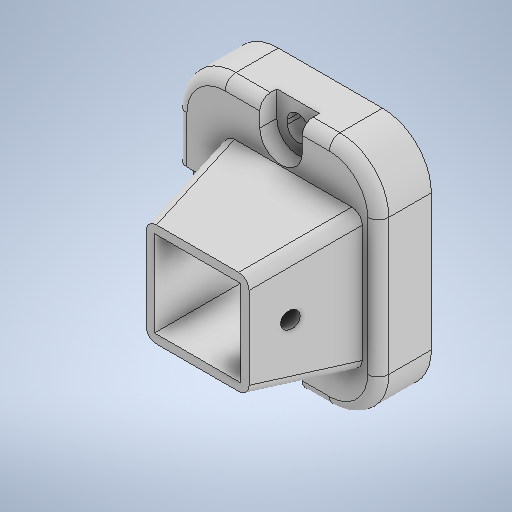
# Autodesk Inventor part: HD - 408 PERFIL ALUMINIO - ANCLAJE BASE DE COLUMNA 40X40
Saved by Autodesk Inventor 2025 (Build 290162000, 162)
## iProperties
Created: 2026-01-26
Part Number: HD - 408 PERFIL ALUMINIO - ANCLAJE BASE DE COLUMNA 40X40
Material: Generic
Document SubType Name: Modeling
Designer: Frank
Density: 1 g/cm^3
Appearance: Default
Author: Frank
Autodesk Inventor part; units mm, degrees
sketch "Sketch1" plane through (0, 0, 0) normal (0, 0, 1) x (1, 0, 0)
  line L0 (-72, 110) -> (-23, 110)
  line L1 (0, 87) -> (0, 23)
  line L2 (-23, 0) -> (-72, 0)
  line L3 (-95, 23) -> (-95, 87)
  arc A0 (-72, 110) -> (-95, 87) centre (-72, 87) ccw
  arc A1 (-95, 23) -> (-72, 0) centre (-72, 23) ccw
  arc A2 (-23, 0) -> (0, 23) centre (-23, 23) ccw
  arc A3 (0, 87) -> (-23, 110) centre (-23, 87) ccw
  point P0 (0, 0)
  point P1 (-95, 110)
  point P2 (0, 0)
  point P3 (0, 110)
  point P4 (-95, 0)
  dimension "d0" = 95
  dimension "d1" = 110
  dimension "d2" = 23
  constraints: 8 end point, 8 point on circle, 8 point on line, 8 tangent, 4 centre point, 3 equal radius, 2 parallel, 1 coincident, 1 horizontal, 1 perpendicular
  measures "d0" distance of point (-95, 110) point (0, 110)
  measures "d1" distance of point (-95, 0) point (-95, 110)
  measures "d2" radius of A0
extrude "Extrusion1" add sketch "Sketch1" against normal blind 25
fillet "Fillet1" radius 5 8 edges at (-47.5, 0, 0) (-6.7365, 6.7365, 0) (0, 55, 0) (-6.7365, 103.2635, 0) (-47.5, 110, 0) (-88.2635, 103.2635, 0) (-95, 55, 0) (-88.2635, 6.7365, 0)
sketch "Sketch2" plane through (0, 0, 0) normal (0, 0, 1) x (1, 0, 0)
  line L0 (-35.7103, 0) -> (-35.7103, 12)
  line L1 (-55.7103, 0) -> (-55.7103, 12)
  arc A0 (-35.7103, 12) -> (-55.7103, 12) centre (-45.7103, 12) ccw
  line L2 (-40.7103, 10) -> (-40.7103, 12)
  line L3 (-50.7103, 10) -> (-50.7103, 12)
  arc A1 (-40.7103, 12) -> (-50.7103, 12) centre (-45.7103, 12) ccw
  arc A2 (-50.7103, 10) -> (-40.7103, 10) centre (-45.7103, 10) ccw
  line L4 (-55.7103, 0) -> (-35.7103, 0)
  line L5 (-23, 0) -> (-72, 0) projected
  point P0 (0, 0)
  point P1 (-45.7103, 22)
  point P2 (-45.7103, 17)
  point P3 (-45.7103, 5)
  dimension "d5" = 20
  dimension "d9" = 5
  dimension "d11" = 10
  constraints: 10 end point, 9 point on circle, 6 tangent, 3 centre point, 2 vertical, 1 collinear
  measures "d5" distance between parallel lines of L1 L0
  measures "d9" distance of point (-45.71, 22) point (-45.71, 17)
  measures "d11" distance between parallel lines of L2 L3
extrude "Extrusion2" cut sketch "Sketch2" against normal blind 8
sketch "Sketch3" plane through (0, 0, 0) normal (0, 0, 1) x (1, 0, 0)
  line L0 (-40.7103, 10) -> (-40.7103, 12) projected
  line L1 (-40.7103, 12) -> (-40.7103, 10)
  arc A0 (-40.7103, 12) -> (-50.7103, 12) centre (-45.7103, 12) ccw projected
  line L2 (-50.7103, 12) -> (-50.7103, 10) projected
  line L3 (-50.7103, 12) -> (-50.7103, 10)
  arc A1 (-50.7103, 10) -> (-40.7103, 10) centre (-45.7103, 10) ccw projected
  point P0 (0, 0)
  constraints: 4 end point, 1 collinear, 1 vertical
extrude "Extrusion3" cut sketch "Sketch3" against normal through all
ref_plane "Work Plane1" through (-72, 55, -25) normal (0, -1, 0) x (1, 0, 0)
mirror "Mirror1" about plane through (-72, 55, -25) normal (0, -1, 0) of "Extrusion2"
mirror "Mirror2" about plane through (-72, 55, -25) normal (0, -1, 0) of "Extrusion3"
sketch "Sketch5" plane through (0, 0, 0) normal (0, 0, 1) x (1, 0, 0)
  line L0 (-95, 23) -> (-95, 87) projected
  line L1 (-95, 45) -> (-83, 45)
  line L2 (-83, 65) -> (-95, 65)
  line L3 (-95, 65) -> (-95, 45)
  line L4 (19, 55) -> (-114, 55) projected
  arc A0 (-83, 45) -> (-83, 65) centre (-83, 55) ccw
  line L5 (-83, 60) -> (-85, 60)
  line L6 (-85, 50) -> (-83, 50)
  arc A1 (-83, 50) -> (-83, 60) centre (-83, 55) ccw
  arc A2 (-85, 60) -> (-85, 50) centre (-85, 55) ccw
  line L7 (-90, 23) -> (-90, 87) projected
  point P0 (0, 0)
  point P1 (-73, 55)
  point P2 (-78, 55)
  point P3 (-90, 55)
  dimension "d21" = 20
  dimension "d22" = 10
  dimension "d23" = 10
  dimension "d24" = 5
  dimension "d25" = 5
  dimension "d26" = 5
  dimension "d27" = 12
  constraints: 10 end point, 9 point on circle, 6 tangent, 3 centre point, 2 horizontal, 2 parallel, 1 point on line
  measures "d21" distance between parallel lines of L2 L1
  measures "d22" distance between parallel lines of L1 L4
  measures "d23" distance between parallel lines of L6 L5
  measures "d24" distance between parallel lines of L1 L6
  measures "d25" distance of point (-73, 55) point (-78, 55)
  measures "d26" distance from line of L0 point (-90, 55)
  measures "d27" distance from line of L7 point (-78, 55)
extrude "Extrusion4" cut sketch "Sketch5" against normal blind 8 contours L0 L4 L7 L1 | L0 L2 L7 L4 | L7 A2 L6 A1 L4 A0 L1 | L7 L2 A0 L4 A1 L5 A2
sketch "Sketch6" plane through (0, 0, 0) normal (0, 0, 1) x (1, 0, 0)
  arc A0 (-83, 50) -> (-83, 60) centre (-83, 55) ccw projected
  line L0 (-83, 60) -> (-85, 60) projected
  line L1 (-83, 60) -> (-85, 60)
  line L2 (-85, 50) -> (-83, 50) projected
  line L3 (-83, 50) -> (-85, 50)
  arc A1 (-85, 60) -> (-85, 50) centre (-85, 55) ccw projected
  point P0 (0, 0)
  constraints: 4 end point, 1 collinear, 1 horizontal
extrude "Extrusion5" cut sketch "Sketch6" against normal through all
sketch "Sketch9" plane through (0, 0, 0) normal (0, 0, 1) x (1, 0, 0)
  line L0 (-72.5, 22.5) -> (-7.5, 22.5)
  line L1 (-7.5, 22.5) -> (-7.5, 87.5)
  line L2 (-7.5, 87.5) -> (-72.5, 87.5)
  line L3 (-72.5, 87.5) -> (-72.5, 22.5)
  line L4 (-5, 87) -> (-5, 23) projected
  line L5 (-72, 0) -> (-55.7103, 0) projected
  point P0 (0, 0)
  point P1 (-40, 22.5)
  dimension "d42" = 65
  dimension "d43" = 65
  dimension "d44" = 2.5
  dimension "d45" = 22.5
  constraints: 8 end point, 2 parallel, 1 horizontal, 1 midpoint, 1 perpendicular
  measures "d42" distance of L2.end L0.start
  measures "d43" distance of L0.start L0.end
  measures "d44" distance between parallel lines of L4 L1
  measures "d45" distance from line of L5 point (-40, 22.5)
ref_plane "Work Plane3" through (0, 0, 45) normal (0, 0, 1) x (1, 0, 0)
sketch "Sketch10" plane through (0, 0, 45) normal (0, 0, 1) x (1, 0, 0)
  line L0 (-64.25, 30.75) -> (-15.75, 30.75)
  line L1 (-15.75, 30.75) -> (-15.75, 79.25)
  line L2 (-15.75, 79.25) -> (-64.25, 79.25)
  line L3 (-64.25, 79.25) -> (-64.25, 30.75)
  line L4 (0, 23) -> (0, 87) projected
  line L5 (-35.7103, 0) -> (-55.7103, 0) projected
  line L6 (-55.7103, 110) -> (-35.7103, 110) projected
  line L7 (-95, 45) -> (-95, 65) projected
  point P0 (0, 0)
  dimension "d47" = 48.5
  dimension "d48" = 48.5
  dimension "d51" = 30.75
  dimension "d52" = 30.75
  dimension "d53" = 30.75
  constraints: 8 end point, 2 parallel, 1 horizontal, 1 perpendicular
  measures "d47" distance of L2.end L0.start
  measures "d48" distance of L0.start L0.end
  measures "d51" distance between parallel lines of L5 L0
  measures "d52" distance between parallel lines of L6 L2
  measures "d53" distance between parallel lines of L7 L3
loft "Loft1" add profiles "Sketch9", "Sketch10"
sketch "Sketch11" plane through (-64.25, 30.75, 45) normal (0, 0, 1) x (1, 0, 0)
  line L0 (4, 4) -> (44.5, 4)
  line L1 (44.5, 4) -> (44.5, 44.5)
  line L2 (44.5, 44.5) -> (4, 44.5)
  line L3 (4, 44.5) -> (4, 4)
  line L4 (0, 48.5) -> (0, 0) projected
  line L5 (0, 0) -> (48.5, 0) projected
  point P0 (64.25, -30.75)
  dimension "d58" = 40.5
  dimension "d59" = 40.5
  dimension "d60" = 4
  dimension "d61" = 4
  constraints: 8 end point, 2 parallel, 1 horizontal, 1 perpendicular
  measures "d58" distance of L0.start L0.end
  measures "d59" distance of L2.end L0.start
  measures "d60" distance between parallel lines of L4 L3
  measures "d61" distance between parallel lines of L5 L0
extrude "Extrusion7" cut sketch "Sketch11" against normal blind 45
fillet "Fillet2" radius 5 4 edges at (-11.625, 26.625, 22.5) (-68.375, 26.625, 22.5) (-11.625, 83.375, 22.5) (-68.375, 83.375, 22.5)
ref_plane "Work Plane4" through (-7.5, 27.418, 0) normal (0.9836066, 0, 0.1803279) x (0.1803279, 0, -0.9836066)
sketch "Sketch12" plane through (-7.5, 27.418, 0) normal (0.9836066, 0, 0.1803279) x (0.1803279, 0, -0.9836066)
  circle A0 centre (-29.0574, 28.2593) radius 4
  line L0 (25.9426, 59.582) -> (25.9426, -4.418) projected
  line L1 (-53.7746, 47.832) -> (-46.4713, 47.832) projected
  point P0 (1.3525, -27.418)
  dimension "d66" = 8
  dimension "d67" = 55
  constraints: 1 centre point
  measures "d66" diameter of A0
  measures "d67" distance from line of L0 A0.centre
extrude "Extrusion8" cut sketch "Sketch12" against normal blind 45
thread "Thread1" size "M8x1.25" class "6H" standard "ANSI Metric M Profile" full length
body "Solid1"
